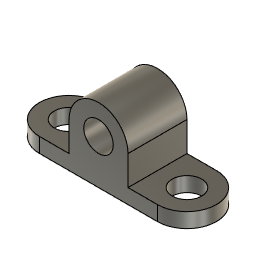
A4 (Autodesk Fusion 360 design; units mm, degrees)
Autodesk Fusion 360 part; units mm, degrees
sketch "Sketch6" plane through (0, 0, 0) normal (0, 0, 1) x (1, 0, 0)
  line L0 (40, -20) -> (-40, -20)
  line L1 (-40, 20) -> (40, 20)
  circle A0 centre (-40, 0) radius 10
  circle A1 centre (40, 0) radius 10
  arc A2 (-40, 20) -> (-40, -20) centre (-40, 0) ccw
  arc A3 (40, -20) -> (40, 20) centre (40, 0) ccw
  dimension "d15" = 80
  dimension "d16" = 40
  constraint horizontal L0
  constraint parallel L0 L1
  measures "d15" distance of L1.start L1.end
  measures "d16" distance of L0.end L1.start
extrude "Extrude4" add sketch "Sketch6" along normal blind 10
sketch "Sketch7" plane through (0, 0, 0) normal (0, 1, 0) x (1, 0, 0)
  line L0 (-20, -10) -> (20, -10)
  line L1 (20, -10) -> (20, -30)
  line L2 (-20, -30) -> (-20, -10)
  circle A0 centre (0, -30) radius 10
  arc A1 (-20, -30) -> (20, -30) centre (0, -30) ccw
  dimension "d22" = 40
  dimension "d23" = 20
  constraint horizontal L0
  constraint vertical L1
  constraint vertical L2
  measures "d22" distance of L0.start L0.end
  measures "d23" distance of L0.start L2.start
extrude "Extrude5" add sketch "Sketch7" along normal mid plane 40
